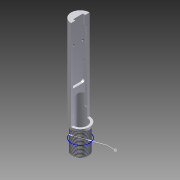
# Autodesk Inventor part: PEEK-PCB-holder
Saved by Autodesk Inventor 2012 (Build 160160000, 160)
## iProperties
Created: 2014-06-23
Part Number: PEEK-PCB-holder
Material: Polyaryletherketon-Kunststoff
Document SubType Name: Modeling
Designer: kathrin.ganzhorn
Density: 1.32 g/cm^3
Mass: 0.946631 g
Surface Area: 20.3493 cm^2
Volume: 0.717145 cm^3
Author: kathrin.ganzhorn
Autodesk Inventor part; units mm, degrees
ref_plane "XZ Plane" through (0, 0, 0) normal (0, 1, 0) x (-1, 0, 0)
ref_plane "XY Plane" through (0, 0, 0) normal (0, 0, 1) x (1, 0, 0)
sketch "Skizze1" plane through (0, 0, 0) normal (0, 0, 1) x (1, 0, 0)
  circle A0 centre (0, 0) radius 4
  dimension "d0" = 8
  constraints: 1 centre point, 1 coincident
  measures "d0" diameter of A0
extrude "Extrusion1" add sketch "Skizze1" along normal blind 45
ref_plane "Mittelebene" through (0, 0, 0) normal (1, 0, 0) x (0, 1, 0)
ref_plane "Mittelebene - PCB-Dicke" through (-1, 0, 0) normal (1, 0, 0) x (0, 1, 0)
sketch "Skizze8" plane through (0, 0, 0) normal (1, 0, 0) x (0, 1, 0)
  line L0 (-4, 45) -> (4, 45)
  line L1 (4, 45) -> (4, 6)
  line L2 (4, 6) -> (-4, 6)
  line L3 (-4, 6) -> (-4, 45)
  point P0 (0, 0)
  dimension "d100" = 8
  dimension "d101" = 39
  constraints: 8 end point, 2 parallel, 1 horizontal, 1 perpendicular
  measures "d100" distance of L1.end L2.end
  measures "d101" distance of L0.end L1.end
extrude "Extrusion6" cut sketch "Skizze8" along normal blind 14.5
sketch "Skizze12" plane through (-1, 0, 0) normal (1, 0, 0) x (0, 1, 0)
  line L0 (2.1, 10) -> (-2.1, 10)
  line L1 (-2.1, 10) -> (-2.1, 45)
  line L2 (-2.1, 45) -> (2.1, 45)
  line L3 (2.1, 45) -> (2.1, 10)
  point P0 (0, 0)
  dimension "d103" = 4.2
  dimension "d104" = 35
  constraints: 8 end point, 2 parallel, 1 horizontal, 1 perpendicular
  measures "d103" distance of L1.end L2.end
  measures "d104" distance of L0.end L1.end
extrude "Extrusion8" cut sketch "Skizze12" along normal blind 6.75
sketch "Skizze13" plane through (-1, 0, 0) normal (1, 0, 0) x (0, 1, 0)
  line L0 (3.1, 10) -> (-3.1, 10)
  line L1 (-3.1, 10) -> (-3.1, 41.2)
  line L2 (-3.1, 41.2) -> (3.1, 41.2)
  line L3 (3.1, 41.2) -> (3.1, 10)
  point P0 (0, 0)
  dimension "d105" = 6.2
  dimension "d106" = 31.2
  constraints: 8 end point, 2 parallel, 1 horizontal, 1 perpendicular
  measures "d105" distance of L1.end L2.end
  measures "d106" distance of L0.end L1.end
extrude "Extrusion9" cut sketch "Skizze13" along normal blind 6.25
sketch "Skizze14" plane through (-1, 0, 0) normal (1, 0, 0) x (0, 1, 0)
  point P0 (0, 0)
  point P1 (-2, 35)
  point P2 (2, 35)
hole "Bohrung3" at (-1, -2, 35) at (-1, 2, 35) direction (-1, 0, 0) diameter 1 end through all
thread "Gewinde5" size "M1x0.25" class "6H" standard "ANSI Metric M Profile" full length
thread "Gewinde6" size "M1x0.25" class "6H" standard "ANSI Metric M Profile" full length
sketch "Skizze15" plane through (0, 0, 0) normal (0, 0, -1) x (-1, 0, 0)
  circle A0 centre (0, 0) radius 4
  dimension "d78" = 8
  constraints: 1 centre point
  measures "d78" diameter of A0
extrude "Extrusion12" add sketch "Skizze15" along normal blind 5
hole "Bohrung5" at (0, 0, 0) direction (0, 0, -1) diameter 6 end through all
hole "Bohrung6" at (0, 0, 0) direction (0, 0, 1) diameter 6 depth 15 tip angle 118
sketch "Skizze16" plane through (0, 0, -5) normal (0, 0, -1) x (-1, 0, 0)
  circle A0 centre (0, 0) radius 4 projected
  circle A1 centre (0, 0) radius 3.5
  dimension "d95" = 7
  constraints: 1 centre point, 1 coincident
  measures "d95" diameter of A1
extrude "Extrusion13" cut sketch "Skizze16" against normal blind 10
thread "Gewinde7" size "M7x0.5" class "6g" standard "ANSI Metric M Profile" length 10
fillet "Rundung1" radius 1 1 edges at (-0.5, -3.1, 41.2)
fillet "Rundung2" radius 1 1 edges at (-0.5, 3.1, 41.2)
sketch "Skizze17" plane through (-1, 0, 0) normal (1, 0, 0) x (0, 0, -1)
  line L0 (-19, -3) -> (-28, -3)
  line L1 (-28, -3) -> (-28, 3)
  line L2 (-28, 3) -> (-19, 3)
  line L3 (-19, 3) -> (-19, -3)
  point P0 (0, 0)
  dimension "d114" = 9
  dimension "d115" = 6
  constraints: 8 end point, 2 parallel, 1 horizontal, 1 perpendicular
  measures "d114" distance of L1.end L2.end
  measures "d115" distance of L0.end L1.end
extrude "Extrusion14" cut sketch "Skizze17" against normal blind 1
fillet "Rundung6" radius 1 4 edges at (-1.5, -3, 19) (-1.5, 3, 19) (-1.5, 3, 28) (-1.5, -3, 28)
